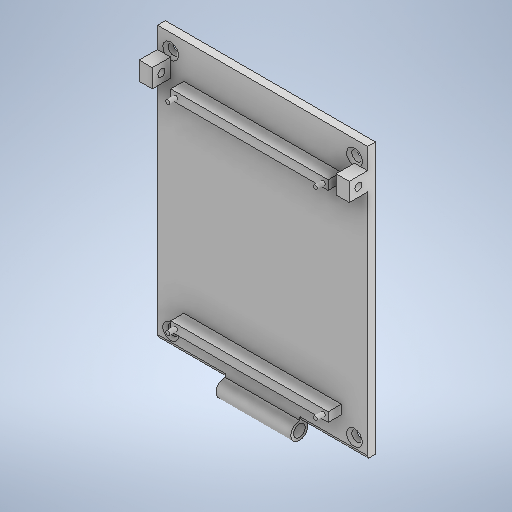
# Autodesk Inventor part: Backboard deel 1
Saved by Autodesk Inventor 2025.2 (Build 292293000, 293)
## iProperties
Created: 2024-12-12
Part Number: Backboard deel 1
Material: Generic
Document SubType Name: Modeling
Designer: jurre
Density: 1 g/cm^3
Appearance: Default
Author: jurre
Autodesk Inventor part; units mm, degrees
ref_plane "YZ Plane" through (0, 0, 0) normal (1, 0, 0) x (0, 1, 0)
ref_plane "XZ Plane" through (0, 0, 0) normal (0, 1, 0) x (-1, 0, 0)
ref_plane "XY Plane" through (0, 0, 0) normal (0, 0, 1) x (1, 0, 0)
sketch "Sketch1" plane through (0, 0, 0) normal (0, 0, 1) x (1, 0, 0)
  line L0 (25.0097, 21.6893) -> (25.0097, -77.3107)
  line L1 (25.0097, -77.3107) -> (-54.9903, -77.3107)
  line L2 (-54.9903, -77.3107) -> (-54.9903, 21.6893)
  line L3 (-44.9903, 12.6893) -> (15.0097, 12.6893)
  line L4 (15.0097, 12.6893) -> (15.0097, -67.3107)
  line L5 (15.0097, -67.3107) -> (-44.9903, -67.3107)
  line L6 (-44.9903, -67.3107) -> (-44.9903, 12.6893)
  circle A0 centre (13.1097, 10.7893) radius 0.75
  circle A1 centre (-43.0903, 10.7893) radius 0.75
  circle A2 centre (-43.0903, -65.4107) radius 0.75
  circle A3 centre (13.1097, -65.4107) radius 0.75
  line L7 (-44.9903, 12.6893) -> (15.0097, 12.6893)
  line L8 (15.0097, 12.6893) -> (15.0097, 9.1893)
  line L9 (15.0097, 9.1893) -> (-44.9903, 9.1893)
  line L10 (-44.9903, 9.1893) -> (-44.9903, 12.6893)
  line L11 (15.0097, -67.3107) -> (-44.9903, -67.3107)
  line L12 (-44.9903, -67.3107) -> (-44.9903, -63.8107)
  line L13 (-44.9903, -63.8107) -> (15.0097, -63.8107)
  line L14 (15.0097, -63.8107) -> (15.0097, -67.3107)
  circle A4 centre (-49.9903, 20.1893) radius 2
  circle A5 centre (20.0097, 20.1893) radius 2
  circle A6 centre (20.0097, -72.3107) radius 2
  circle A7 centre (-49.9903, -72.3107) radius 2
  line L15 (-54.9903, 26.1893) -> (25.0097, 26.1893)
  line L16 (25.0097, 26.1893) -> (25.0097, -77.3107)
  line L17 (25.0097, -77.3107) -> (-54.9903, -77.3107)
  line L18 (-54.9903, -77.3107) -> (-54.9903, 26.1893)
  line L19 (-54.9903, 18.1893) -> (-49.9903, 18.1893)
  line L20 (-49.9903, 18.1893) -> (-49.9903, 11.1893)
  line L21 (-49.9903, 11.1893) -> (-54.9903, 11.1893)
  line L22 (-54.9903, 11.1893) -> (-54.9903, 18.1893)
  line L23 (25.0097, 18.1893) -> (20.0097, 18.1893)
  line L24 (20.0097, 18.1893) -> (20.0097, 11.1893)
  line L25 (20.0097, 11.1893) -> (25.0097, 11.1893)
  line L26 (25.0097, 11.1893) -> (25.0097, 18.1893)
  point P0 (0, 0)
  point P1 (-14.9903, -77.3107)
  point P2 (-44.9903, 9.1893)
  point P3 (15.0097, 9.1893)
  point P4 (15.0097, -63.8107)
  point P5 (-44.9903, -63.8107)
  point P6 (25.0097, 11.1893)
  point P7 (25.0097, 18.1893)
  point P8 (-54.9903, 18.1893)
  point P9 (-54.9903, 11.1893)
  dimension "d4" = 10
  dimension "d5" = 10
  dimension "d6" = 1.5
  dimension "d7" = 1.5
  dimension "d8" = 1.5
  dimension "d9" = 1.5
  dimension "d11" = 1.9
  dimension "d12" = 1.9
  dimension "d13" = 1.9
  dimension "d14" = 1.9
  dimension "d15" = 1.9
  dimension "d16" = 1.9
  dimension "d17" = 1.9
  dimension "d18" = 1.9
  dimension "d20" = 0
  dimension "d21" = 0
  dimension "d22" = 3.5
  dimension "d24" = 0
  dimension "d25" = 3.5
  dimension "d26" = 0
  dimension "d39" = 4
  dimension "d41" = 5
  dimension "d42" = 4
  dimension "d43" = 4
  dimension "d44" = 4
  dimension "d46" = 5
  dimension "d47" = 5
  dimension "d48" = 5
  dimension "d49" = 5
  dimension "d50" = 5
  dimension "d70" = 80
  dimension "d71" = 103.5
  dimension "d75" = 6
  dimension "d76" = 5
  dimension "d77" = 7
  dimension "d78" = 5
  dimension "d79" = 7
  dimension "d91" = 8
  dimension "d92" = 8
  dimension "d97" = 60
  dimension "d105" = 80
  constraints: 54 end point, 13 parallel, 8 centre point, 6 horizontal, 6 perpendicular, 2 point on line, 1 midpoint
  measures "d4" distance from line of point (-14.99, -77.311) L5
  measures "d5" distance between parallel lines of L0 L4
  measures "d6" diameter of A0
  measures "d7" diameter of A1
  measures "d8" diameter of A2
  measures "d9" diameter of A3
  measures "d11" distance from line of L3 A1.centre
  measures "d12" distance from line of L6 A1.centre
  measures "d13" distance from line of L3 A0.centre
  measures "d14" distance from line of L4 A0.centre
  measures "d15" distance from line of L4 A3.centre
  measures "d16" distance from line of L5 A3.centre
  measures "d17" distance from line of L6 A2.centre
  measures "d18" distance from line of L5 A2.centre
  measures "d20" distance between parallel lines of L4 L8
  measures "d21" distance between parallel lines of L3 L7
  measures "d22" distance of L9.end L7.start
  measures "d24" distance between parallel lines of L4 L14
  measures "d25" distance of L13.end L11.start
  measures "d26" distance between parallel lines of L5 L11
  measures "d39" diameter of A4
  measures "d41" distance from line of L2 A4.centre
  measures "d42" diameter of A5
  measures "d43" diameter of A6
  measures "d44" diameter of A7
  measures "d46" distance from line of L0 A5.centre
  measures "d47" distance from line of L0 A6.centre
  measures "d48" distance from line of L1 A6.centre
  measures "d49" distance from line of L2 A7.centre
  measures "d50" distance from line of L1 A7.centre
  measures "d70" distance of L15.start L15.end
  measures "d71" distance of L15.end L0.end
  measures "d75" distance from line of L15 A5.centre
  measures "d76" distance of L20.end L21.end
  measures "d77" distance of L19.end L20.end
  measures "d78" distance of L24.end L25.end
  measures "d79" distance of L23.end L24.end
  measures "d91" distance between parallel lines of L23 L15
  measures "d92" distance between parallel lines of L19 L15
  measures "d97" distance of L8.end L9.end
  measures "d105" distance of L3.end L4.end
extrude "Extrusion5" add sketch "Sketch1" against normal blind 3 contours A4 | A5 | L0 L23 L24 L25 L1 L2 L21 L20 L19 L18 L15 L16 | L0 L25 L24 L23 | L19 L20 L21 L2 | L3 L4 L9 L6 | L9 L4 L13 L6 | L13 L4 L5 L6 | A0 | A1 | A2 | A3 | A6 | A7
extrude "Extrusion7" add sketch "Sketch1" along normal blind 5 contours L3 L4 L9 L6 | L13 L4 L5 L6 | A0 | A1 | A2 | A3
extrude "Extrusion8" add sketch "Sketch1" along normal blind 8 contours A0 | A1 | A2 | A3
sketch "Sketch3" plane through (25.0097, -77.3107, -3) normal (1, 0, 0) x (0, 0, -1)
  circle A0 centre (-3.25, -3) radius 3.25
  line L0 (-3, 0) -> (0, 0) projected
  line L1 (-3, 0) -> (-3, 103.5) projected
  circle A1 centre (-3.25, -3) radius 2.25
  line L2 (0, 103.5) -> (0, 0) projected
  point P0 (-3, 77.3107)
  point P1 (-3, 99)
  point P2 (0, 100)
  point P3 (-3, 100)
  dimension "d60" = 6.5
  dimension "d61" = 3
  dimension "d63" = 4.5
  dimension "d64" = 3.25
  constraints: 2 centre point, 1 coincident
  measures "d60" diameter of A0
  measures "d61" distance from line of L0 A0.centre
  measures "d63" diameter of A1
  measures "d64" distance from line of L2 A0.centre
extrude "Extrusion9" add sketch "Sketch3" along normal blind 28.5 separate body
move or copy body "Move Body1" bodies to move or copy 2 copy no translate (-54.25, 0, 0)
combine bodies "Combine1" operation type add bodies to combine 1 2
extrude "Extrusion10" add sketch "Sketch1" against normal blind 3 contours A4 | A5 | L0 L23 L24 L25 L1 L2 L21 L20 L19 L18 L15 L16 | L0 L25 L24 L23 | L19 L20 L21 L2 | L3 L4 L9 L6 | L9 L4 L13 L6 | L13 L4 L5 L6 | A0 | A1 | A2 | A3 | A6 | A7 bodies 1
extrude "Extrusion11" cut sketch "Sketch1" against normal blind 4 contours A4 | A5 | A6 | A7 bodies 1
fillet "Fillet3" radius 1 4 edges at (-51.9903, 20.1893, 0) (18.0097, 20.1893, 0) (18.0097, -72.3107, 0) (-51.9903, -72.3107, 0)
extrude "Extrusion12" add sketch "Sketch1" along normal blind 7 contours L0 L25 L24 L23 | L19 L20 L21 L2 bodies 1
sketch "Sketch4" plane through (25.0097, -77.3107, -3) normal (1, 0, 0) x (0, 0, -1)
  circle A0 centre (-6.5, 92) radius 1.375
  line L0 (-10, 88.5) -> (-10, 95.5) projected
  line L1 (-3, 95.5) -> (-10, 95.5) projected
  line L2 (-3, 88.5) -> (-10, 88.5) projected
  point P0 (-3, 77.3107)
  dimension "d85" = 2.75
  dimension "d86" = 3.5
  dimension "d87" = 3.5
  dimension "d88" = 3.5
  constraints: 1 centre point
  measures "d85" diameter of A0
  measures "d86" distance from line of A0.centre L0
  measures "d87" distance from line of A0.centre L1
  measures "d88" distance from line of L2 A0.centre
extrude "Extrusion13" cut sketch "Sketch4" against normal blind 200 bodies 1
sketch "Sketch5" plane through (-0.7403, -77.3107, 0) normal (1, 0, 0) x (0, 0, -1)
  line L0 (0, 0) -> (3, 0) projected
  arc A0 (0, 0.2404) -> (1, 0) centre (-0.25, -3) ccw projected
  line L1 (3, 0) -> (3, -3)
  line L2 (0, 0) -> (3, -3)
  line L3 (0, 0) -> (3, 0)
  point P0 (0, 77.3107)
  constraints: 6 end point, 1 collinear, 1 point on circle, 1 vertical
extrude "Extrusion14" add sketch "Sketch5" against normal blind 28.5 bodies 1
fillet "Fillet4" radius 1.5 2 edges at (12.1347, -77.3107, 0) (-42.1153, -77.3107, 0)
sketch "Sketch6" plane through (25.0097, -77.3107, -3) normal (1, 0, 0) x (0, 0, -1)
  line L0 (0, 0) -> (-1.5, 0) projected
  line L1 (-3, 1.5) -> (-3, 0.2404) projected
  line L2 (0, 0) -> (-3, 0)
  line L3 (-3, 0) -> (-3, 0.5)
  line L4 (-3, 0.5) -> (0, 0.5)
  line L5 (0, 0.5) -> (0, 0)
  point P0 (-3, 77.3107)
  point P1 (-3, 0.2404)
  point P2 (-1.5, 0)
  dimension "d99" = 0.5
  constraints: 8 end point, 2 parallel, 1 horizontal, 1 perpendicular, 1 point on line
  measures "d99" distance of L2.end L3.end
extrude "Extrusion15" cut sketch "Sketch6" against normal blind 25.75 bodies 1
sketch "Sketch7" plane through (-54.9903, -77.3107, -3) normal (-1, 0, 0) x (0, 0, 1)
  line L0 (0, 0) -> (1.5, 0) projected
  line L1 (3, 0.2404) -> (3, 1.5) projected
  line L2 (0, 0) -> (3, 0)
  line L3 (3, 0) -> (3, 0.5)
  line L4 (3, 0.5) -> (0, 0.5)
  line L5 (0, 0.5) -> (0, 0)
  point P0 (3, 77.3107)
  point P1 (1.5, 0)
  point P2 (3, 0.2404)
  dimension "d102" = 0.5
  constraints: 8 end point, 2 parallel, 1 horizontal, 1 perpendicular, 1 point on line
  measures "d102" distance of L2.end L3.end
extrude "Extrusion16" cut sketch "Sketch7" against normal blind 25.75 bodies 1
equation "\"d80\" = d43"
body "Solid2"
